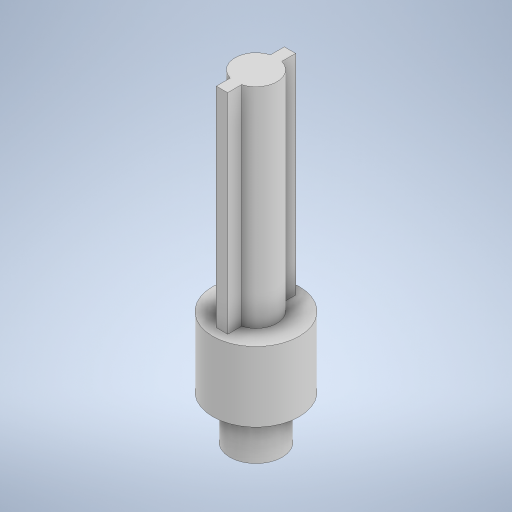
# Autodesk Inventor part: spojkaMotoruSRotorem
Saved by Autodesk Inventor 2023 (Build 270158000, 158)
## iProperties
Created: 2023-11-08
Part Number: spojkaMotoruSRotorem
Material: Generic
Document SubType Name: Modeling
Designer: alexa
Density: 1 g/cm^3
Appearance: Default
Author: alexa
Autodesk Inventor part; units mm, degrees
ref_plane "YZ Plane" through (0, 0, 0) normal (1, 0, 0) x (0, 1, 0)
ref_plane "XZ Plane" through (0, 0, 0) normal (0, 1, 0) x (-1, 0, 0)
ref_plane "XY Plane" through (0, 0, 0) normal (0, 0, 1) x (1, 0, 0)
sketch "Sketch1" plane through (0, 0, 0) normal (0, 1, 0) x (-1, 0, 0)
  circle A0 centre (0, 0) radius 4.95
  dimension "d0" = 9.9
  constraints: 1 centre point, 1 coincident
  measures "d0" diameter of A0
extrude "Extrusion1" add sketch "Sketch1" along normal blind 8
sketch "Sketch2" plane through (0, 8, 0) normal (0, 1, 0) x (1, 0, 0)
  circle A0 centre (0, 0) radius 2.4
  line L0 (-0.65, -3.9) -> (0.65, -3.9)
  line L1 (0.65, -3.9) -> (0.65, 3.9)
  line L2 (0.65, 3.9) -> (-0.65, 3.9)
  line L3 (-0.65, 3.9) -> (-0.65, -3.9)
  line L4 (-0.65, -3.9) -> (0.65, 3.9) construction
  line L5 (0.65, -3.9) -> (-0.65, 3.9) construction
  point P0 (-0.65, 2.3103)
  point P1 (-0.65, -2.3103)
  point P2 (0.65, -2.3103)
  point P3 (0.65, 2.3103)
  dimension "d3" = 4.8
  dimension "d4" = 1.3
  dimension "d5" = 7.8
  constraints: 12 end point, 2 midpoint, 2 parallel, 1 centre point, 1 coincident, 1 horizontal, 1 perpendicular
  measures "d3" diameter of A0
  measures "d4" distance of L1.end L2.end
  measures "d5" distance of L2.end L0.start
extrude "Extrusion2" add sketch "Sketch2" along normal blind 24
sketch "Sketch3" plane through (0, 0, 0) normal (0, -1, 0) x (1, 0, 0)
  circle A0 centre (0, 0) radius 3
  dimension "d8" = 6
  constraints: 1 centre point, 1 coincident
  measures "d8" diameter of A0
extrude "Extrusion3" add sketch "Sketch3" along normal blind 5
sketch "Sketch4" plane through (0, -5, 0) normal (0, -1, 0) x (1, 0, 0)
  arc A0 (-0.65, 2.3103) -> (-0.65, -2.3103) centre (0, 0) ccw projected
  circle A1 centre (0, 0) radius 1.75
  line L0 (1.3857, -0.85) -> (-1.5, -0.85)
  line L1 (1.3857, -0.85) -> (1.8275, -0.85)
  line L2 (-1.5, -0.85) -> (-1.5752, -0.85)
  point P0 (-0.5831, -1.65)
  point P1 (0.5831, -1.65)
  point P2 (1.5297, -0.85)
  point P3 (-1.5297, -0.85)
  dimension "d11" = 3.5
  dimension "d12" = 2.6
  constraints: 6 end point, 3 horizontal, 1 centre point, 1 coincident
  measures "d11" diameter of A1
extrude "Extrusion6" cut sketch "Sketch4" against normal blind 10 contours A1 L1 L0 L2 picked at (-0.5593, -0.3047)
body "Solid1"
